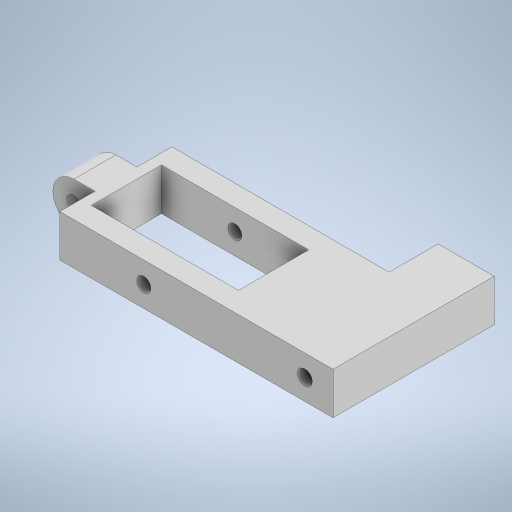
# Autodesk Inventor part: drzak_pritlacneho_kolecka
Saved by Autodesk Inventor 2023.1 (Build 271208000, 208)
## iProperties
Created: 2023-01-11
Part Number: drzak_pritlacneho_kolecka
Material: Generic
Document SubType Name: Modeling
Designer: zavrel
Density: 1 g/cm^3
Appearance: Default
Author: zavrel
Autodesk Inventor part; units mm, degrees
ref_plane "YZ Plane" through (0, 0, 0) normal (1, 0, 0) x (0, 1, 0)
ref_plane "XZ Plane" through (0, 0, 0) normal (0, 1, 0) x (-1, 0, 0)
sketch "Sketch1" plane through (0, 0, 0) normal (0, 1, 0) x (-1, 0, 0)
  line L0 (0, 0) -> (18.1846, 0) construction
  line L1 (0, 0) -> (0, 15)
  line L2 (0, 15) -> (8, 15)
  line L3 (8, 15) -> (8, 8)
  line L4 (8, 8) -> (39, 8)
  line L5 (39, 8) -> (39, 3)
  line L6 (39, 3) -> (45, 3)
  line L7 (45, 3) -> (45, 0)
  line L8 (0, 0) -> (0, -15)
  line L9 (0, -15) -> (8, -15)
  line L10 (8, -15) -> (8, -8)
  line L11 (8, -8) -> (39, -8)
  line L12 (39, -8) -> (39, -3)
  line L13 (39, -3) -> (45, -3)
  line L14 (45, -3) -> (45, 0)
  point P0 (45, 1.5)
  dimension "d0" = 6
  dimension "d1" = 45
  dimension "d2" = 8
  dimension "d3" = 8
  dimension "d4" = 15
  dimension "d5" = 3
  constraints: 30 end point, 6 perpendicular, 6 symmetric about line, 1 horizontal, 1 midpoint, 1 point on line, 1 vertical
  measures "d0" distance of L5.end L6.end
  measures "d1" distance from line of point (45, 1.5) L1
  measures "d2" distance between parallel lines of L1 L3
  measures "d3" distance from line of L0.start L4
  measures "d4" distance from line of L0.start L2
  measures "d5" distance from line of L7.end L6
extrude "Extrusion1" add sketch "Sketch1" along normal blind 6
sketch "Sketch2" plane through (-39, 0, -3) normal (0, 0, -1) x (-1, 0, 0)
  line L0 (0, 0) -> (6, 0) projected
  line L1 (6, 0) -> (6, 6) projected
  line L2 (0, 6) -> (6, 6) projected
  line L3 (0, 0) -> (0, 6) projected
  circle A0 centre (3, 3) radius 1
  point P0 (-39, 0)
  point P1 (6, 3)
  dimension "d8" = 3
  dimension "d9" = 2
  constraints: 1 centre point, 1 horizontal alignment, 1 midpoint
  measures "d8" distance from line of L1 A0.centre
  measures "d9" diameter of A0
extrude "Extrusion2" cut sketch "Sketch2" against normal blind 6 contours A0
sketch "Sketch3" plane through (0, 6, 0) normal (0, 1, 0) x (1, 0, 0)
  line L0 (-8, 15) -> (-8, 8) projected
  line L1 (-8, 8) -> (-39, 8) projected
  line L2 (-39, 8) -> (-39, 3) projected
  line L3 (-39, 3) -> (-45, 3) projected
  line L4 (-45, 3) -> (-45, -3) projected
  line L5 (-45, -3) -> (-39, -3) projected
  line L6 (-39, -3) -> (-39, -8) projected
  line L7 (-39, -8) -> (-8, -8) projected
  line L8 (-8, -8) -> (-8, -15) projected
  line L9 (-8, -15) -> (0, -15) projected
  line L10 (0, -15) -> (0, 15) projected
  line L11 (0, 15) -> (-8, 15) projected
  line L12 (-45, 3) -> (-45, -3) construction
  line L13 (-45, 0) -> (0, 0) construction
  line L14 (-16.5, -5) -> (-37.5, -5)
  line L15 (-37.5, -5) -> (-37.5, 5)
  line L16 (-37.5, 5) -> (-16.5, 5)
  line L17 (-16.5, 5) -> (-16.5, -5)
  point P0 (-42, -3)
  point P1 (-27, -5)
  dimension "d12" = 10
  dimension "d13" = 21
  dimension "d14" = 15
  constraints: 10 end point, 3 midpoint, 2 horizontal, 2 parallel, 1 perpendicular, 1 other
  measures "d12" distance of L14.end L15.end
  measures "d13" distance of L14.start L14.end
  measures "d14" horizontal distance of point (-42, -3) point (-27, -5)
extrude "Extrusion3" cut sketch "Sketch3" against normal through all contours L14 L15 L16 L17
sketch "Sketch4" plane through (-8, 0, -8) normal (0, 0, -1) x (-1, 0, 0)
  line L0 (29.5, 0) -> (8.5, 0) projected
  line L1 (29.5, 6) -> (29.5, 0) projected
  line L2 (8.5, 6) -> (29.5, 6) projected
  line L3 (8.5, 6) -> (8.5, 0) projected
  circle A0 centre (19, 3) radius 1
  point P0 (-8, 0)
  point P1 (10.5, 6)
  point P2 (29.5, 3)
  point P3 (19, 6)
  dimension "d17" = 2
  constraints: 2 midpoint, 1 centre point, 1 horizontal alignment, 1 vertical alignment
  measures "d17" diameter of A0
extrude "Extrusion4" cut sketch "Sketch4" against normal through all contours A0
fillet "Fillet1" radius 3 2 edges at (-45, 6, 0) (-45, 0, 0)
sketch "Náčrt5" plane through (0, 0, -15) normal (0, 0, -1) x (-1, 0, 0)
  line L0 (0, 0) -> (8, 0) projected
  line L1 (8, 0) -> (8, 6) projected
  line L2 (0, 6) -> (8, 6) projected
  line L3 (0, 0) -> (0, 6) projected
  circle A0 centre (4, 3) radius 1.05
  point P0 (0, 0)
  point P1 (8, 3)
  point P2 (4, 6)
  dimension "d21" = 2.1
  constraints: 2 midpoint, 1 centre point, 1 horizontal alignment, 1 vertical alignment
  measures "d21" diameter of A0
extrude "Vysunutí5" cut sketch "Náčrt5" against normal through all contours A0
ref_plane "Pracovní rovina1" through (0, 0, 0) normal (0, 0, -1) x (-1, 0, 0)
sketch "Sketch9" plane through (0, 0, 0) normal (0, -1, 0) x (1, 0, 0)
  line L0 (-42, -3) -> (-42, 3) projected
  line L1 (-39, -3) -> (-42, -3) projected
  line L2 (-39, -8) -> (-39, -3) projected
  line L3 (-8, -8) -> (-39, -8) projected
  line L4 (-8, -15) -> (-8, -8) projected
  line L5 (0, -15) -> (-8, -15) projected
  line L6 (0, 15) -> (0, -15) projected
  line L7 (-8, 15) -> (0, 15) projected
  line L8 (-8, 8) -> (-8, 15) projected
  line L9 (-39, 8) -> (-8, 8) projected
  line L10 (-39, 3) -> (-39, 8) projected
  line L11 (-42, 3) -> (-39, 3) projected
  line L12 (-16.5, -5) -> (-37.5, -5) projected
  line L13 (-37.5, -5) -> (-37.5, 5) projected
  line L14 (-37.5, 5) -> (-16.5, 5) projected
  line L15 (-16.5, 5) -> (-16.5, -5) projected
  line L16 (-2.95, -15) -> (-5.05, -15) projected
  line L17 (-1.8376, -6.4564) -> (-6.1624, -6.4564)
  line L18 (-6.1624, -6.4564) -> (-6.1624, -12.5436)
  line L19 (-6.1624, -12.5436) -> (-1.8376, -12.5436)
  line L20 (-1.8376, -12.5436) -> (-1.8376, -6.4564)
  line L21 (0, -15) -> (-8, -15) construction
  line L22 (-4, -15) -> (-4, 15) construction
  line L23 (-8, 15) -> (0, 15) construction
  point P0 (0, 0)
  point P1 (0, 0)
  point P2 (-1.8376, -9.5)
  dimension "d29" = 9.5
  constraints: 10 end point, 4 midpoint, 2 parallel, 1 horizontal, 1 perpendicular, 1 other
  measures "d29" vertical distance of point (0, 0) point (-1.838, -9.5)
extrude "Extrusion7" cut sketch "Sketch9" against normal blind 5 contours L20 L19 L18 L17
sketch "Sketch10" plane through (0, 0, 0) normal (0, -1, 0) x (1, 0, 0)
  line L0 (-1.8376, -12.5436) -> (-6.1624, -12.5436) projected
  line L1 (-6.1624, -12.5436) -> (-6.1624, -6.4564) projected
  line L2 (-6.1624, -6.4564) -> (-1.8376, -6.4564) projected
  line L3 (-1.8376, -6.4564) -> (-1.8376, -12.5436) projected
  line L4 (-42, -3) -> (-42, 3) projected
  line L5 (-39, -3) -> (-42, -3) projected
  line L6 (-39, -8) -> (-39, -3) projected
  line L7 (-8, -8) -> (-39, -8) projected
  line L8 (-8, -15) -> (-8, -8) projected
  line L9 (0, -15) -> (-8, -15) projected
  line L10 (0, 15) -> (0, -15) projected
  line L11 (-8, 15) -> (0, 15) projected
  line L12 (-8, 8) -> (-8, 15) projected
  line L13 (-39, 8) -> (-8, 8) projected
  line L14 (-39, 3) -> (-39, 8) projected
  line L15 (-42, 3) -> (-39, 3) projected
  line L16 (-37.5, -5) -> (-37.5, 5) projected
  line L17 (-37.5, 5) -> (-16.5, 5) projected
  line L18 (-16.5, 5) -> (-16.5, -5) projected
  line L19 (-16.5, -5) -> (-37.5, -5) projected
  line L20 (-8, 8) -> (-8, 15) projected
  line L21 (-8, 8) -> (0, 8)
  point P0 (0, 0)
  constraints: 2 end point, 1 perpendicular, 1 point on line
extrude "Extrusion8" cut sketch "Sketch10" against normal through all contours L12 L11 L10 L21
body "Solid1"
